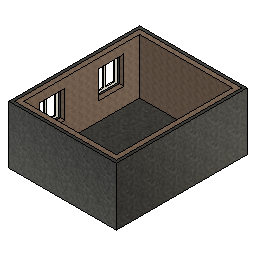
Pièce climaitsée (Autodesk Fusion 360 design; units mm, degrees)
Autodesk Fusion 360 part; units mm, degrees
sketch "Esquisse1" plane through (0, 0, 0) normal (0, 0, 1) x (1, 0, 0)
  line L0 (0, 0) -> (4000, 0)
  line L1 (4000, 0) -> (4000, 5000)
  line L2 (4000, 5000) -> (0, 5000)
  line L3 (0, 5000) -> (0, 0)
  line L4 (0, 5000) -> (4000, 5000)
  line L5 (4000, 5000) -> (4000, 5200)
  line L6 (4000, 5200) -> (0, 5200)
  line L7 (0, 5200) -> (0, 5000)
  line L8 (0, 0) -> (4000, 0)
  line L9 (4000, 0) -> (4000, -200)
  line L10 (4000, -200) -> (0, -200)
  line L11 (0, -200) -> (0, 0)
  line L12 (4000, -200) -> (4200, -200)
  line L13 (4200, -200) -> (4200, 5200)
  line L14 (4200, 5200) -> (4000, 5200)
  line L15 (4000, 5200) -> (4000, -200)
  line L16 (0, -200) -> (-200, -200)
  line L17 (-200, -200) -> (-200, 5200)
  line L18 (-200, 5200) -> (0, 5200)
  line L19 (0, 5200) -> (0, -200)
  line L20 (-200, 5200) -> (4200, 5200)
  line L21 (4200, 5200) -> (4200, 5320)
  line L22 (4200, 5320) -> (-200, 5320)
  line L23 (-200, 5320) -> (-200, 5200)
  line L24 (-200, -200) -> (4200, -200)
  line L25 (4200, -200) -> (4200, -320)
  line L26 (4200, -320) -> (-200, -320)
  line L27 (-200, -320) -> (-200, -200)
  line L28 (-200, 5320) -> (-320, 5320)
  line L29 (-320, 5320) -> (-320, -320)
  line L30 (-320, -320) -> (-200, -320)
  line L31 (-200, -320) -> (-200, 5320)
  line L32 (4200, 5320) -> (4320, 5320)
  line L33 (4320, 5320) -> (4320, -320)
  line L34 (4320, -320) -> (4200, -320)
  line L35 (4200, -320) -> (4200, 5320)
  dimension "d1" = 4000
  dimension "d4" = 5000
  dimension "d5" = 200
  dimension "d6" = 120
  dimension "d7" = 120
  dimension "d8" = 120
  dimension "d9" = 120
  dimension "d11" = 200
  constraint horizontal L0
  constraint vertical L1
  constraint horizontal L2
  constraint vertical L3
  constraint coincident L0.start L3.end
  constraint horizontal L4
  constraint vertical L5
  constraint horizontal L6
  constraint vertical L7
  constraint horizontal L8
  constraint vertical L9
  constraint horizontal L10
  constraint vertical L11
  constraint horizontal L12
  constraint vertical L13
  constraint horizontal L14
  constraint vertical L15
  constraint horizontal L16
  constraint vertical L17
  constraint horizontal L18
  constraint vertical L19
  constraint horizontal L20
  constraint vertical L21
  constraint horizontal L22
  constraint vertical L23
  constraint horizontal L24
  constraint vertical L25
  constraint horizontal L26
  constraint vertical L27
  constraint horizontal L28
  constraint vertical L29
  constraint horizontal L30
  constraint vertical L31
  constraint horizontal L32
  constraint vertical L33
  constraint horizontal L34
  constraint vertical L35
  constraint collinear L26 L34
  constraint collinear L26 L30
  constraint collinear L6 L20
  measures "d1" distance of L0.start L0.end
  measures "d4" distance of L0.end L1.end
  measures "d5" distance of L2.end L6.end
  measures "d6" distance of L17.end L22.end
  measures "d7" distance of L16.end L26.end
  measures "d8" distance of L22.end L28.end
  measures "d9" distance of L21.end L32.end
  measures "d11" distance of L0 L10
extrude "Extrusion1" add sketch "Esquisse1" along normal blind 1 contours L0 L1 L2 L3 L4 L8 L15 L19 makes body 1
extrude "Extrusion3" add sketch "Esquisse1" along normal blind 2500 separate body contours L10 L12 L16 L24 L25 L26 L27 L31 L35 | L6 L14 L18 L20 L21 L22 L23 L31 L35 | L17 L23 L27 L28 L29 L30 L31 | L13 L21 L25 L32 L33 L34 L35 makes body 2
extrude "Extrusion4" add 1 faces at (1333.3333, 3333.3333, 1) along direction (0, 0, 1) blind 120 separate body on bodies 1 makes body 3
extrude "Extrusion2" add sketch "Esquisse1" along normal blind 2500 separate body contours L3 L7 L11 L16 L17 L18 L19 L20 L24 L31 | L0 L8 L9 L10 L11 L15 L19 L24 | L1 L5 L9 L12 L13 L14 L15 L20 L24 L35 | L2 L4 L5 L6 L7 L15 L19 L20 makes body 4
sketch "Esquisse2" plane through (-320, 0, 0) normal (-1, 0, 0) x (0, -1, 0)
  line L0 (-5320, 0) -> (320, 0)
  line L1 (320, 0) -> (320, 2500)
  line L2 (320, 2500) -> (-5320, 2500)
  line L3 (-5320, 2500) -> (-5320, 0)
  line L4 (-1780, 2100) -> (-680, 2100)
  line L5 (-680, 2100) -> (-680, 900)
  line L6 (-680, 900) -> (-1780, 900)
  line L7 (-1780, 900) -> (-1780, 2100)
  line L8 (-5320, 0) -> (320, 0)
  line L9 (-4320, 2100) -> (-3220, 2100)
  line L10 (-3220, 2100) -> (-3220, 900)
  line L11 (-3220, 900) -> (-4320, 900)
  line L12 (-4320, 900) -> (-4320, 2100)
  dimension "d18" = 900
  dimension "d19" = 1100
  dimension "d20" = 1200
  dimension "d21" = 1100
  dimension "d22" = 1200
  dimension "d23" = 900
  dimension "d24" = 1000
  dimension "d25" = 1000
  constraint horizontal L4
  constraint vertical L5
  constraint horizontal L6
  constraint vertical L7
  constraint horizontal L9
  constraint vertical L10
  constraint horizontal L11
  constraint vertical L12
  measures "d18" distance of L6 L8
  measures "d19" distance of L4.start L4.end
  measures "d20" distance of L4.end L5.end
  measures "d21" distance of L9.start L9.end
  measures "d22" distance of L9.start L11.end
  measures "d23" distance of L8 L11
  measures "d24" distance of L1 L5
  measures "d25" distance of L3 L12
extrude "Extrusion5" cut sketch "Esquisse2" against normal up to surface (320 mm away) contours L4 L5 L6 L7 | L9 L10 L11 L12 bodies 2 4
sketch "Esquisse1 (2)" plane through (-320, 0, 0) normal (-1, 0, 0) x (0, -1, 0) in component "Fenetre"
  line L0 (-4320, 900) -> (-4320, 2100)
  line L1 (-4320, 2100) -> (-3220, 2100)
  line L2 (-3220, 2100) -> (-3220, 900)
  line L3 (-3220, 900) -> (-4320, 900)
  line L4 (-1780, 900) -> (-1780, 2100)
  line L5 (-1780, 2100) -> (-680, 2100)
  line L6 (-680, 2100) -> (-680, 900)
  line L7 (-680, 900) -> (-1780, 900)
  line L8 (-5320, 0) -> (320, 0)
  line L9 (320, 0) -> (320, 2500)
  line L10 (320, 2500) -> (-5320, 2500)
  line L11 (-5320, 2500) -> (-5320, 0)
  line L12 (-4320, 2100) -> (-3220, 2100)
  line L13 (-3220, 2100) -> (-3220, 900)
  line L14 (-3220, 900) -> (-4320, 900)
  line L15 (-4320, 900) -> (-4320, 2100)
  line L16 (-4200, 2000) -> (-3300, 2000)
  line L17 (-3300, 2000) -> (-3300, 1000)
  line L18 (-3300, 1000) -> (-4200, 1000)
  line L19 (-4200, 1000) -> (-4200, 2000)
  line L20 (-3800, 2000) -> (-3700, 2000)
  line L21 (-3700, 2000) -> (-3700, 1000)
  line L22 (-3700, 1000) -> (-3800, 1000)
  line L23 (-3800, 1000) -> (-3800, 2000)
  constraint horizontal L12
  constraint vertical L13
  constraint horizontal L14
  constraint vertical L15
  constraint coincident L2.end L3.start
  constraint coincident L0.end L1.start
  constraint horizontal L16
  constraint vertical L17
  constraint horizontal L18
  constraint vertical L19
  constraint horizontal L20
  constraint vertical L21
  constraint horizontal L22
  constraint vertical L23
  constraint coincident L18 L21.end
  constraint coincident L16 L20.start
extrude "Extrusion1'" add sketch "Esquisse1 (2)" against normal blind 50 separate body contours L0 L1 L2 L3 L12 L13 L14 L15 | L16 L18 L20 L21 L22 L23 makes body 5 in component "Fenetre"
component "Fenetre" placed x (1, 0, 0) y (0, 1, 0) z (0, 0, 1) at (0, 0, 0)
component "Fenetre" placed x (1, 0, 0) y (0, 1, 0) z (0, 0, 1) at (0, -2545, 0)
equation "d23 = d18"
equation "d25 = d24"
named bodies: "Dalle", "IsolationMurs", "IsolationSol", "Murs"
